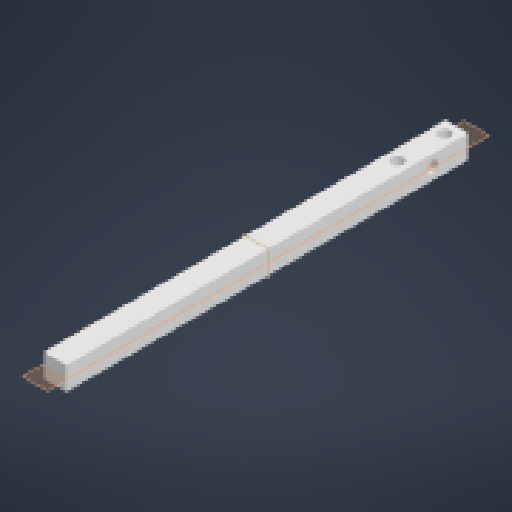
# Autodesk Inventor part: Part5
Saved by Autodesk Inventor 2026 (Build 300175000, 175)
## iProperties
Created: 2025-10-09
Part Number: Part5
Material: Generic
Document SubType Name: Modeling
Designer: kenny
Density: 1 g/cm^3
Appearance: Default
Author: kenny
Autodesk Inventor part; units mm, degrees
ref_plane "YZ Plane" through (0, 0, 0) normal (1, 0, 0) x (0, 1, 0)
ref_plane "XZ Plane" through (0, 0, 0) normal (0, 1, 0) x (-1, 0, 0)
ref_plane "XY Plane" through (0, 0, 0) normal (0, 0, 1) x (1, 0, 0)
sketch "Sketch1" plane through (0, 0, 0) normal (0, 0, 1) x (1, 0, 0)
  line L0 (0, 0) -> (7.8, 0)
  line L1 (7.8, 0) -> (7.8, 7.8)
  line L2 (7.8, 7.8) -> (0, 7.8)
  line L3 (0, 7.8) -> (0, 0)
  dimension "d0" = 7.8
  dimension "d1" = 7.8
  constraints: 8 end point, 2 parallel, 1 horizontal, 1 perpendicular
  measures "d0" distance of L2.end L1.end
  measures "d1" distance of L1.end L0.end
extrude "Extrusion1" add sketch "Sketch1" along normal blind 136
sketch "Sketch2" plane through (0, 7.8, 0) normal (0, 1, 0) x (1, 0, 0)
  line L0 (0, 0) -> (3.9, 0)
  line L1 (7.8, 0) -> (0, 0) projected
  line L2 (3.9, 0) -> (3.9, -2.2)
  line L3 (3.9, -2.2) -> (3.9, -4.2)
  circle A0 centre (3.9, -4.2) radius 2
  dimension "d4" = 2.2
  dimension "d5" = 2
  dimension "d6" = 4
  constraints: 6 end point, 1 centre point, 1 coincident, 1 midpoint, 1 perpendicular, 1 point on line
  measures "d4" distance of L0.end L2.end
  measures "d5" distance of L2.end L3.end
  measures "d6" diameter of A0
extrude "Extrusion2" cut sketch "Sketch2" against normal blind 136
sketch "Sketch3" plane through (7.8, 0, 0) normal (1, 0, 0) x (0, 0, -1)
  line L0 (0, 0) -> (0, 7.8) projected
  line L1 (0, 7.8) -> (0, 3.9)
  line L2 (0, 3.9) -> (-10.2, 3.9)
  line L3 (-10.2, 3.9) -> (-12.2, 3.9)
  circle A0 centre (-12.2, 3.9) radius 2
  dimension "d9" = 10.2
  dimension "d10" = 2
  constraints: 6 end point, 1 coincident, 1 horizontal alignment, 1 midpoint, 1 perpendicular, 1 point on line, 2 other
  measures "d9" distance of L1.end L2.end
  measures "d10" distance of L2.end L3.end
extrude "Extrusion3" cut sketch "Sketch3" against normal blind 136
sketch "Sketch4" plane through (0, 7.8, 0) normal (0, 1, 0) x (1, 0, 0)
  circle A0 centre (3.9, -4.2) radius 2 projected
  line L0 (3.9, -6.2) -> (3.9, -8.4)
  line L1 (0, 0) -> (7.8, 0) projected
  line L2 (7.8, -10.2) -> (0, -10.2) projected
  line L3 (3.9, -8.4) -> (3.9, -10.4)
  line L4 (3.9, -6.2) -> (3.9, -18.2)
  line L5 (3.9, -18.2) -> (3.9, -20.2)
  circle A1 centre (3.9, -20.2) radius 2
  dimension "d13" = 2.2
  dimension "d15" = 2
  dimension "d16" = 12
  dimension "d17" = 2
  constraints: 8 end point, 2 vertical, 2 vertical alignment, 1 coincident, 1 perpendicular, 1 point on line, 3 other
  measures "d13" distance of L0.start L0.end
  measures "d15" distance of L0.end L3.end
  measures "d16" distance of L0.start L4.end
  measures "d17" distance of L4.end L5.end
extrude "Extrusion4" cut sketch "Sketch4" against normal blind 136 contours A1
ref_plane "Work Plane1" through (0, 0, 68) normal (0, 0, -1) x (-1, 0, 0)
ref_plane "Work Plane2" through (0, 3.9, 0) normal (0, 1, 0) x (1, 0, 0)
body "Solid1"
